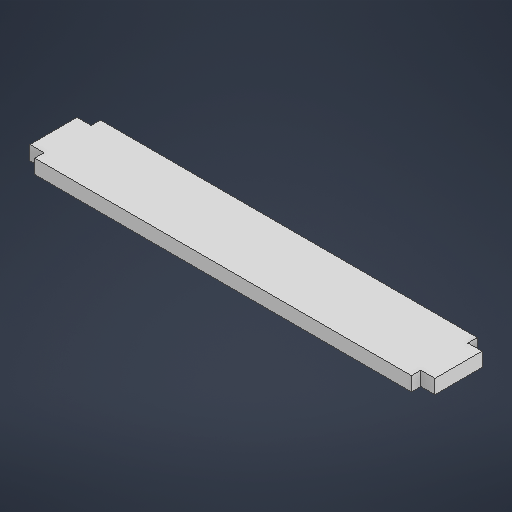
# Autodesk Inventor part: soporte_base_parqueo
Saved by Autodesk Inventor 2026 (Build 300175000, 175)
## iProperties
Created: 2026-05-15
Part Number: soporte_base_parqueo
Material: Generic
Document SubType Name: Modeling
Designer: juana
Density: 1 g/cm^3
Appearance: Default
Author: juana
Autodesk Inventor part; units mm, degrees
ref_plane "YZ Plane" through (0, 0, 0) normal (1, 0, 0) x (0, 1, 0)
ref_plane "XZ Plane" through (0, 0, 0) normal (0, 1, 0) x (-1, 0, 0)
ref_plane "XY Plane" through (0, 0, 0) normal (0, 0, 1) x (1, 0, 0)
sketch "Sketch1" plane through (0, 0, 0) normal (0, 1, 0) x (-1, 0, 0)
  line L0 (0, 0) -> (80, 0)
  line L1 (80, 0) -> (80, -14)
  line L2 (80, -14) -> (0, -14)
  line L3 (0, -14) -> (0, 0)
  line L4 (80, -2) -> (83, -2)
  line L5 (83, -2) -> (83, -12)
  line L6 (83, -12) -> (80, -12)
  line L7 (40, -14) -> (40, 0) construction
  line L8 (0, -2) -> (-3, -2)
  line L9 (-3, -2) -> (-3, -12)
  line L10 (-3, -12) -> (0, -12)
  dimension "d0" = 14
  dimension "d1" = 80
  dimension "d2" = 2
  dimension "d3" = 10
  dimension "d4" = 3
  constraints: 22 end point, 4 symmetric about line, 3 perpendicular, 2 horizontal, 2 midpoint, 2 parallel, 2 point on line
  measures "d0" distance of L0.end L1.end
  measures "d1" distance of L1.end L2.end
  measures "d2" distance between parallel lines of L0 L4
  measures "d3" distance of L4.end L5.end
  measures "d4" distance of L5.end L6.end
extrude "Extrusion1" add sketch "Sketch1" along normal blind 3
body "Solid1"
